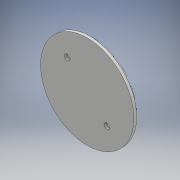
# Autodesk Inventor part: WifiPixels
Saved by Autodesk Inventor 2018 (Build 220112000, 112)
## iProperties
Created: 2017-07-21
Part Number: WifiPixels
Material: Generic
Document SubType Name: Modeling
Designer: Micha
Density: 1 g/cm^3
Appearance: Default
Author: Micha
Autodesk Inventor part; units mm, degrees
ref_plane "YZ Plane" through (0, 0, 0) normal (1, 0, 0) x (0, 1, 0)
ref_plane "XZ Plane" through (0, 0, 0) normal (0, 1, 0) x (-1, 0, 0)
ref_plane "XY Plane" through (0, 0, 0) normal (0, 0, 1) x (1, 0, 0)
sketch "Sketch1" plane through (0, 0, 0) normal (0, 1, 0) x (-1, 0, 0)
  circle A0 centre (0, 0) radius 25
  line L0 (0, 0) -> (10.6066, 10.6066)
  line L1 (0, 0) -> (15, 0) construction
  circle A1 centre (10.6066, 10.6066) radius 1.5
  line L2 (0, 0) -> (-10.6066, -10.6066)
  line L3 (0, 0) -> (15, 0) construction
  circle A2 centre (-10.6066, -10.6066) radius 1.5
  dimension "d0" = 50
  dimension "d1" = 15
  dimension "d2" = 45
  dimension "d3" = 3
  dimension "d4" = 15
  dimension "d5" = 135
  dimension "d6" = 3
  constraints: 8 end point, 3 centre point, 3 coincident, 2 equal length, 2 horizontal
  measures "d0" diameter of A0
  measures "d1" distance of L0.start L0.end
  measures "d2" angle of L1 L0
  measures "d3" diameter of A1
  measures "d4" distance of L0.start L2.end
  measures "d5" angle of L2 L3
  measures "d6" diameter of A2
extrude "Extrusion1" add sketch "Sketch1" along normal blind 1.5
sketch "Sketch2" plane through (0, 1.5, 0) normal (0, 1, 0) x (1, 0, 0)
  line L0 (0, 0) -> (-23.5, 0)
  line L1 (0, 0) -> (23.5, 0) construction
  line L2 (-23.5, 0) -> (-23.5, 2.5)
  line L3 (-23.5, 2.5) -> (-18.5, 2.5)
  line L4 (-18.5, 2.5) -> (-18.5, -2.5)
  line L5 (-18.5, -2.5) -> (-23.5, -2.5)
  line L6 (-23.5, -2.5) -> (-23.5, 2.5)
  dimension "d9" = 23.5
  dimension "d10" = 180
  dimension "d11" = 2.5
  dimension "d12" = 90
  dimension "d13" = 5
  dimension "d14" = 5
  constraints: 14 end point, 3 horizontal, 2 parallel, 2 perpendicular, 1 collinear
  measures "d9" distance of L0.start L0.end
  measures "d10" angle of L0 L1
  measures "d11" distance of L0.end L2.end
  measures "d12" angle of L0 L2
  measures "d13" distance of L4.end L5.end
  measures "d14" distance of L3.end L4.end
extrude "Extrusion2" add sketch "Sketch2" along normal blind 1.5
pattern_circular "Circular Pattern1" count 16 over 360 about axis through (0, 0, 0) along (0, 1, 0) of "Extrusion2"
body "Solid1"
